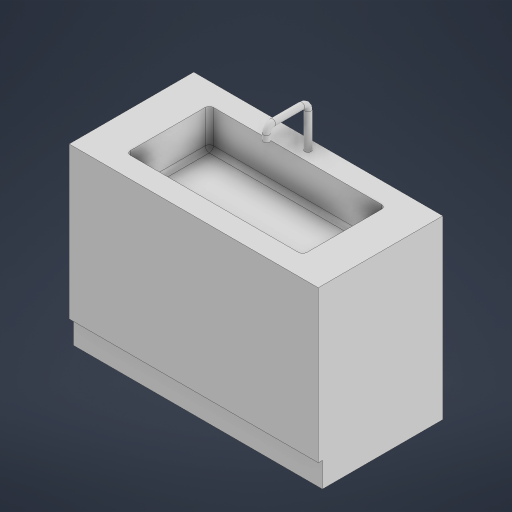
# Autodesk Inventor part: Mobile lavandino 1200
Saved by Autodesk Inventor 2024.2 (Build 282272000, 272)
## iProperties
Created: 2025-08-13
Part Number: Mobile lavandino 1200
Material: Generic
Document SubType Name: Modeling
Designer: Luca
Density: 1 g/cm^3
Appearance: Default
Author: Luca
Autodesk Inventor part; units mm, degrees
ref_plane "YZ Plane" through (0, 0, 0) normal (1, 0, 0) x (0, 1, 0)
ref_plane "XZ Plane" through (0, 0, 0) normal (0, 1, 0) x (-1, 0, 0)
ref_plane "XY Plane" through (0, 0, 0) normal (0, 0, 1) x (1, 0, 0)
sketch "Sketch1" plane through (0, 0, 0) normal (0, 1, 0) x (-1, 0, 0)
  line L0 (600, 0) -> (-600, 0)
  line L1 (-600, 0) -> (-600, 600)
  line L2 (-600, 600) -> (600, 600)
  line L3 (600, 600) -> (600, 0)
  point P0 (0, 0)
  point P1 (0, 0)
  dimension "d0" = 1200
  dimension "d1" = 600
  constraints: 8 end point, 2 parallel, 1 coincident, 1 horizontal, 1 midpoint, 1 perpendicular
  measures "d0" distance of L1.end L2.end
  measures "d1" distance of L0.end L1.end
extrude "Extrusion1" add sketch "Sketch1" along normal blind 850
sketch "Sketch2" plane through (0, 850, 0) normal (0, 1, 0) x (1, 0, 0)
  line L0 (-425, -500) -> (425, -500)
  line L1 (425, -500) -> (425, -100)
  line L2 (425, -100) -> (-425, -100)
  line L3 (-425, -100) -> (-425, -500)
  line L4 (-425, -500) -> (425, -100) construction
  line L5 (425, -500) -> (-425, -100) construction
  line L6 (-600, 0) -> (-600, -600) projected
  line L7 (-600, -600) -> (600, -600) projected
  point P0 (0, 0)
  point P1 (0, -300)
  point P2 (-600, -300)
  point P3 (-600, -300)
  point P4 (0, -600)
  dimension "d4" = 850
  dimension "d5" = 400
  constraints: 12 end point, 5 midpoint, 2 parallel, 1 horizontal, 1 horizontal alignment, 1 perpendicular, 1 vertical alignment
  measures "d4" distance of L2.end L1.end
  measures "d5" distance of L1.end L0.end
extrude "Extrusion2" cut sketch "Sketch2" against normal blind 180
fillet "Fillet1" radius 20 8 edges at (-425, 760, 100) (-425, 670, 300) (0, 670, 100) (-425, 760, 500) (0, 670, 500) (425, 670, 300) (425, 760, 500) (425, 760, 100)
sketch "Sketch3" plane through (-600, 0, 600) normal (0, 0, 1) x (1, 0, 0)
  line L0 (0, 0) -> (1200, 0) projected
  line L1 (1200, 0) -> (1200, 850) projected
  line L2 (0, 0) -> (1200, 0)
  line L3 (1200, 0) -> (1200, 120)
  line L4 (1200, 120) -> (0, 120)
  line L5 (0, 120) -> (0, 0)
  point P0 (600, 0)
  dimension "d9" = 120
  constraints: 8 end point, 2 parallel, 1 horizontal, 1 perpendicular, 1 point on line
  measures "d9" distance of L3.end L2.end
extrude "Extrusion3" cut sketch "Sketch3" against normal blind 20
sketch "Sketch4" plane through (0, 0, 0) normal (1, 0, 0) x (0, 1, 0)
  line L0 (850, 120) -> (850, 100) projected
  line L1 (850, 120) -> (850, 480) projected
  line L2 (850, 500) -> (850, 480) projected
  line L3 (850, 480) -> (850, 500) projected
  line L4 (850, 480) -> (850, 120) projected
  line L5 (850, 100) -> (850, 120) projected
  line L6 (850, 600) -> (850, 0) projected
  line L7 (850, 0) -> (850, 600) projected
  line L8 (850, 50) -> (1020, 50)
  arc A0 (1020, 50) -> (1050, 80) centre (1020, 80) ccw
  line L9 (1050, 80) -> (1050, 220)
  arc A1 (1050, 220) -> (1020, 250) centre (1020, 220) ccw
  line L10 (1020, 250) -> (990, 250)
  point P0 (0, 0)
  dimension "d12" = 60
  dimension "d13" = 200
  dimension "d14" = 50
  dimension "d15" = 200
  dimension "d16" = 30
  constraints: 6 end point, 4 point on circle, 4 tangent, 3 perpendicular, 2 centre point, 1 equal radius, 1 point on line
  measures "d12" distance from line of L10.end L9
  measures "d13" distance between parallel lines of L8 L10
  measures "d14" distance from line of L6.end L8
  measures "d15" distance between parallel lines of L6 L9
  measures "d16" radius of A0
sketch "Sketch5" plane through (0, 850, 0) normal (0, 1, 0) x (1, 0, 0)
  circle A0 centre (0, -50) radius 15
  point P0 (0, 0)
  dimension "d17" = 30
  constraints: 1 centre point, 1 coincident
  measures "d17" diameter of A0
sweep "Sweep1" add profiles "Sketch5" path "Sketch4" path curves L8 A0 L9 A1 L10
body "Solid1"
